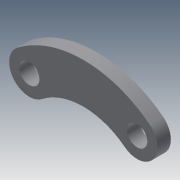
# Autodesk Inventor part: tahlo-neco_sablona
Saved by Autodesk Inventor 2013 (Build 170138000, 138)
## iProperties
Created: 2013-06-14
Part Number: tahlo-neco_sablona
Material: Generic
Document SubType Name: Modeling
Designer: idle-rug
Density: 1 g/cm^3
Author: idle-rug
Autodesk Inventor part; units mm, degrees
ref_plane "YZ Plane" through (0, 0, 0) normal (1, 0, 0) x (0, 1, 0)
ref_plane "XZ Plane" through (0, 0, 0) normal (0, 1, 0) x (-1, 0, 0)
ref_plane "XY Plane" through (0, 0, 0) normal (0, 0, 1) x (1, 0, 0)
sketch "Sketch1" plane through (0, 0, 0) normal (0, 1, 0) x (-1, 0, 0)
  circle A0 centre (8, 0) radius 3
  line L0 (8, 0) -> (-8, 0)
  circle A1 centre (-8, 0) radius 3
  arc A2 (6.1538, -2.3647) -> (-6.1538, -2.3647) centre (0, -10.247) ccw
  line L1 (0, -0.247) -> (0, 5.753)
  arc A3 (9.8462, 2.3647) -> (-9.8462, 2.3647) centre (0, -10.247) ccw
  circle A4 centre (8, 0) radius 1.5
  circle A5 centre (-8, 0) radius 1.5
  point P0 (0, 0)
  dimension "d13" = 16
  dimension "d14" = 6
  dimension "d16" = 6
  dimension "d17" = 3
  dimension "d18" = 3
  constraints: 10 point on circle, 6 centre point, 4 end point, 3 coincident, 1 horizontal, 1 perpendicular, 1 other
  measures "d13" distance of L0.start L0.end
  measures "d14" diameter of A1
  measures "d16" distance of L1.start L1.end
  measures "d17" diameter of A4
  measures "d18" diameter of A5
extrude "Extrusion1" add sketch "Sketch1" along normal blind 2
body "Solid1"
